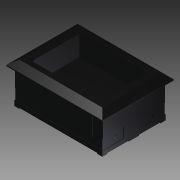
# Autodesk Inventor part: UB16NKG015F-NR
Saved by Autodesk Inventor 2015 SP1 (Build 190203100, 203)
## iProperties
Category: Electrical
Company: Autodesk Inc.
Created: 2014-12-16
Part Number: UB16NKG015F-NR
Catalog Web Link: http://www.nkkswitches.com/
Description: UB_ill_body-Illuminated Pushbuttons - Series UB
Vendor: NKK Switches
Document SubType Name: Modeling
Designer: Autodesk Inc.
Manufacturer: NKKSWITCHES
Mass: 2.33276 g
Surface Area: 18.6541 cm^2
Volume: 2.33276 cm^3
Density: 1 g/cm^3
Material: Generic
Appearance: PSOLRGB-0-0-0
PSOL_IDENT_2: ION=},{LINEID=10},{LINESUBID=-1},{WBVAR=PLS,MT}  {NB=UB1NK-body_},{LINA=UB1NK-body_},{KT=DUMMY},{SRS=
PSOL_IDENT_3: UB},{PLS=1},{MT=NK}
SUPPLIER: NKKSWITCHES
Title: UB1NK-body_
Author: Autodesk Inc.
Comments: Illuminated Pushbuttons - Series UB
Autodesk Inventor part; units mm, degrees
sketch "Sketch_2" plane through (0, 0, 0) normal (0, 0, 1) x (1, 0, 0)
  line L0 (-12.0015, 8.6106) -> (-10.9982, 8.6106)
  line L1 (-10.9982, 8.6106) -> (-10.9982, 3.81)
  line L2 (-10.9982, 3.81) -> (-10.8712, 3.81)
  line L3 (-10.8712, 3.81) -> (-10.8712, 1.27)
  line L4 (-10.8712, 1.27) -> (-10.9982, 1.27)
  line L5 (-10.9982, 1.27) -> (-10.9982, 0)
  line L6 (-10.9982, 0) -> (10.9982, 0)
  line L7 (10.9982, 0) -> (10.9982, 1.27)
  line L8 (10.9982, 1.27) -> (10.8712, 1.27)
  line L9 (10.8712, 1.27) -> (10.8712, 3.81)
  line L10 (10.8712, 3.81) -> (10.9982, 3.81)
  line L11 (10.9982, 3.81) -> (10.9982, 8.6106)
  line L12 (10.9982, 8.6106) -> (12.0015, 8.6106)
  line L13 (12.0015, 8.6106) -> (12.0015, 8.8646)
  line L14 (12.0015, 8.8646) -> (10.3691, 10.0076)
  line L15 (10.3691, 10.0076) -> (-10.3691, 10.0076)
  line L16 (-10.3691, 10.0076) -> (-12.0015, 8.8646)
  line L17 (-12.0015, 8.8646) -> (-12.0015, 8.6106)
  constraints: 36 end point
extrude "Extrusion1" add sketch "Sketch_2" along normal mid plane 24.003
sketch "Sketch_1" plane through (0, 0, 0) normal (1, 0, 0) x (0, 1, 0)
  line L0 (12.7, 12.7) -> (-2.54, 12.7)
  line L1 (-2.54, 12.7) -> (-2.54, -12.7)
  line L2 (-2.54, -12.7) -> (12.7, -12.7)
  line L3 (12.7, -12.7) -> (12.7, 12.7)
  line L4 (8.6106, 8.9027) -> (8.6106, 7.7724)
  line L5 (8.6106, 7.7724) -> (1.27, 7.7724)
  line L6 (1.27, 7.7724) -> (1.27, 7.8994)
  line L7 (1.27, 7.8994) -> (0, 7.8994)
  line L8 (0, 7.8994) -> (0, -7.8994)
  line L9 (0, -7.8994) -> (1.27, -7.8994)
  line L10 (1.27, -7.8994) -> (1.27, -7.7724)
  line L11 (1.27, -7.7724) -> (8.6106, -7.7724)
  line L12 (8.6106, -7.7724) -> (8.6106, -8.9027)
  line L13 (8.6106, -8.9027) -> (8.8646, -8.9027)
  line L14 (8.8646, -8.9027) -> (10.0076, -7.2703)
  line L15 (10.0076, -7.2703) -> (10.0076, 7.2703)
  line L16 (10.0076, 7.2703) -> (8.8646, 8.9027)
  line L17 (8.8646, 8.9027) -> (8.6106, 8.9027)
  constraints: 36 end point
extrude "Extrusion2" cut sketch "Sketch_1" along normal mid plane 25.4
sketch "Sketch_3" plane through (0, 10.0076, 0) normal (0, 1, 0) x (1, 0, 0)
  line L0 (-8.4963, 5.4864) -> (-8.4963, -5.4864)
  arc A0 (-8.4963, -5.4864) -> (-7.9883, -5.9944) centre (-7.9883, -5.4864) ccw
  line L1 (-7.9883, -5.9944) -> (7.9883, -5.9944)
  arc A1 (7.9883, -5.9944) -> (8.4963, -5.4864) centre (7.9883, -5.4864) ccw
  line L2 (8.4963, -5.4864) -> (8.4963, 5.4864)
  arc A2 (8.4963, 5.4864) -> (7.9883, 5.9944) centre (7.9883, 5.4864) ccw
  line L3 (7.9883, 5.9944) -> (-7.9883, 5.9944)
  arc A3 (-7.9883, 5.9944) -> (-8.4963, 5.4864) centre (-7.9883, 5.4864) ccw
  constraints: 8 end point, 8 point on circle, 4 centre point
sketch "Sketch_4" plane through (0, 0, 0) normal (0, 1, 0) x (-1, 0, 0)
  line L0 (10.9982, -6.6294) -> (10.9982, 6.6294)
  line L1 (10.9982, 6.6294) -> (9.7282, 6.6294)
  line L2 (9.7282, 6.6294) -> (9.7282, 7.8994)
  line L3 (9.7282, 7.8994) -> (-9.7282, 7.8994)
  line L4 (-9.7282, 7.8994) -> (-9.7282, 6.6294)
  line L5 (-9.7282, 6.6294) -> (-10.9982, 6.6294)
  line L6 (-10.9982, 6.6294) -> (-10.9982, 1.27)
  line L7 (-10.9982, 1.27) -> (-9.7282, 1.27)
  line L8 (-9.7282, 1.27) -> (-9.7282, -1.27)
  line L9 (-9.7282, -1.27) -> (-10.9982, -1.27)
  line L10 (-10.9982, -1.27) -> (-10.9982, -6.6294)
  line L11 (-10.9982, -6.6294) -> (-9.7282, -6.6294)
  line L12 (-9.7282, -6.6294) -> (-9.7282, -7.8994)
  line L13 (-9.7282, -7.8994) -> (9.7282, -7.8994)
  line L14 (9.7282, -7.8994) -> (9.7282, -6.6294)
  line L15 (9.7282, -6.6294) -> (10.9982, -6.6294)
  constraints: 32 end point
extrude "Extrusion3" cut sketch "Sketch_4" along normal blind 0.2032
sketch "Sketch_6" plane through (0, 0, 0) normal (0, 1, 0) x (-1, 0, 0)
  line L0 (9.7282, 7.1374) -> (1.27, 7.1374)
  line L1 (1.27, 7.1374) -> (1.27, 7.3914)
  line L2 (1.27, 7.3914) -> (-1.27, 7.3914)
  line L3 (-1.27, 7.3914) -> (-1.27, 7.1374)
  line L4 (-1.27, 7.1374) -> (-9.7282, 7.1374)
  line L5 (-9.7282, 7.1374) -> (-9.7282, -7.1374)
  line L6 (-9.7282, -7.1374) -> (9.7282, -7.1374)
  line L7 (9.7282, -7.1374) -> (9.7282, 7.1374)
  constraints: 16 end point
extrude "Extrusion4" cut sketch "Sketch_6" along normal blind 0.4064
sketch "Sketch_9" plane through (0, 0, 0) normal (1, 0, 0) x (0, 1, 0)
  line L0 (1.27, 2.54) -> (1.27, -2.54)
  line L1 (1.27, -2.54) -> (3.81, -2.54)
  line L2 (3.81, -2.54) -> (3.81, 2.54)
  line L3 (3.81, 2.54) -> (1.27, 2.54)
  constraints: 8 end point
extrude "Extrusion5" add sketch "Sketch_9" along normal mid plane 21.9964
sketch "Sketch_8" plane through (0, 2.54, 0) normal (0, 1, 0) x (1, 0, 0)
  line L0 (-10.9982, -4.5974) -> (-10.7442, -5.3594)
  line L1 (-10.7442, -5.3594) -> (-10.7442, -6.6294)
  line L2 (-10.7442, -6.6294) -> (10.7442, -6.6294)
  line L3 (10.7442, -6.6294) -> (10.7442, -5.3594)
  line L4 (10.7442, -5.3594) -> (10.9982, -4.5974)
  line L5 (10.9982, -4.5974) -> (10.9982, -4.0894)
  line L6 (10.9982, -4.0894) -> (10.7442, -4.0894)
  line L7 (10.7442, -4.0894) -> (10.7442, 4.0894)
  line L8 (10.7442, 4.0894) -> (10.9982, 4.0894)
  line L9 (10.9982, 4.0894) -> (10.9982, 4.5974)
  line L10 (10.9982, 4.5974) -> (10.7442, 5.3594)
  line L11 (10.7442, 5.3594) -> (10.7442, 6.6294)
  line L12 (10.7442, 6.6294) -> (-10.7442, 6.6294)
  line L13 (-10.7442, 6.6294) -> (-10.7442, 5.3594)
  line L14 (-10.7442, 5.3594) -> (-10.9982, 4.5974)
  line L15 (-10.9982, 4.5974) -> (-10.9982, 4.0894)
  line L16 (-10.9982, 4.0894) -> (-10.7442, 4.0894)
  line L17 (-10.7442, 4.0894) -> (-10.7442, -4.0894)
  line L18 (-10.7442, -4.0894) -> (-10.9982, -4.0894)
  line L19 (-10.9982, -4.0894) -> (-10.9982, -4.5974)
  constraints: 40 end point
extrude "Extrusion6" add sketch "Sketch_8" along normal mid plane 0.508
sketch "Sketch_19" plane through (0, 0, 0) normal (0, 0, 1) x (1, 0, 0)
  line L0 (-8.4582, 3.048) -> (8.4582, 3.048)
  line L1 (8.4582, 3.048) -> (8.4582, 8.6868)
  line L2 (8.4582, 8.6868) -> (-8.4582, 8.6868)
  line L3 (-8.4582, 8.6868) -> (-8.4582, 3.048)
  constraints: 8 end point
extrude "Extrusion7" add sketch "Sketch_19" along normal mid plane 15.7988
extrude "Extrusion8" cut sketch "Sketch_3" against normal blind 5.08
ref_plane "D_XY" through (0, 0, 0) normal (0, 1, 0) x (1, 0, 0)
ref_plane "D_YZ" through (0, 0, 0) normal (1, 0, 0) x (0, 0, -1)
ref_plane "D_ZX" through (0, 0, 0) normal (0, 0, -1) x (0, 1, 0)
ref_plane "LENS_XY" through (0, 10.0076, 0) normal (0, -1, 0) x (1, 0, 0)
ref_plane "LENS_YZ" through (0, 10.0076, 0) normal (1, 0, 0) x (0, 0, 1)
ref_plane "LENS_ZX" through (0, 10.0076, 0) normal (0, 0, 1) x (0, -1, 0)
ref_plane "P_1_XY" through (7.62, 0.4064, 5.08) normal (0, 1, 0) x (1, 0, 0)
ref_plane "P_1_YZ" through (7.62, 0.4064, 5.08) normal (1, 0, 0) x (0, 0, -1)
ref_plane "P_1_ZX" through (7.62, 0.4064, 5.08) normal (0, 0, -1) x (0, 1, 0)
ref_plane "P_2_XY" through (7.62, 0.4064, 0) normal (0, 1, 0) x (1, 0, 0)
ref_plane "P_2_YZ" through (7.62, 0.4064, 0) normal (1, 0, 0) x (0, 0, -1)
ref_plane "P_2_ZX" through (7.62, 0.4064, 0) normal (0, 0, -1) x (0, 1, 0)
ref_plane "P_3_XY" through (7.62, 0.4064, -5.08) normal (0, 1, 0) x (1, 0, 0)
ref_plane "P_3_YZ" through (7.62, 0.4064, -5.08) normal (1, 0, 0) x (0, 0, -1)
ref_plane "P_3_ZX" through (7.62, 0.4064, -5.08) normal (0, 0, -1) x (0, 1, 0)
ref_plane "P_4_XY" through (0, 0.4064, 2.54) normal (0, 1, 0) x (1, 0, 0)
ref_plane "P_4_YZ" through (0, 0.4064, 2.54) normal (1, 0, 0) x (0, 0, -1)
ref_plane "P_4_ZX" through (0, 0.4064, 2.54) normal (0, 0, -1) x (0, 1, 0)
ref_plane "P_5_XY" through (0, 0.4064, -2.54) normal (0, 1, 0) x (1, 0, 0)
ref_plane "P_5_YZ" through (0, 0.4064, -2.54) normal (1, 0, 0) x (0, 0, -1)
ref_plane "P_5_ZX" through (0, 0.4064, -2.54) normal (0, 0, -1) x (0, 1, 0)
ref_plane "body_to_metal_1_XY" through (0, 0, 0) normal (0, -1, 0) x (1, 0, 0)
ref_plane "body_to_metal_1_YZ" through (0, 0, 0) normal (1, 0, 0) x (0, 0, 1)
ref_plane "body_to_metal_1_ZX" through (0, 0, 0) normal (0, 0, 1) x (0, -1, 0)
ref_plane "body_to_metal_2_XY" through (0, 0, 0) normal (0, -1, 0) x (1, 0, 0)
ref_plane "body_to_metal_2_YZ" through (0, 0, 0) normal (1, 0, 0) x (0, 0, 1)
ref_plane "body_to_metal_2_ZX" through (0, 0, 0) normal (0, 0, 1) x (0, -1, 0)
body "Solid1"
